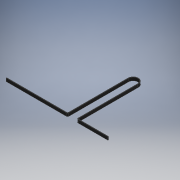
# Autodesk Inventor part: HeaderSliderBelt
Saved by Autodesk Inventor 2017 (Build 210142000, 142)
## iProperties
Created: 2016-12-13
Part Number: HeaderSliderBelt
Material: Rubber
Document SubType Name: Modeling
Designer: umr
Density: 0.93 g/cm^3
Appearance: Rubber - Black
Author: umr
Autodesk Inventor part; units mm, degrees
ref_plane "YZ Plane" through (0, 0, 0) normal (1, 0, 0) x (0, 1, 0)
ref_plane "XZ Plane" through (0, 0, 0) normal (0, 1, 0) x (-1, 0, 0)
ref_plane "XY Plane" through (0, 0, 0) normal (0, 0, 1) x (1, 0, 0)
sketch "Sketch1" plane through (0, 0, 0) normal (0, 0, 1) x (1, 0, 0)
  line L0 (0, 0) -> (99.0465, 0)
  line L1 (98.0465, 0.9998) -> (0.0465, 0.9998)
  line L2 (0.0465, 0.9998) -> (0, 0)
  line L3 (100.0262, 0) -> (101.0465, 0)
  line L4 (101.0465, 2) -> (101.0465, 100)
  line L5 (100.0465, 100) -> (100.0465, 2.9998)
  line L6 (116.9623, 98.8064) -> (116.9623, 3)
  line L7 (116.735, 0) -> (116.0465, 0.7253)
  line L8 (116.0465, 2) -> (116.0465, 100)
  arc A0 (116.9623, 98.8064) -> (100.0465, 100) centre (108.5465, 100) ccw
  arc A1 (116.0465, 100) -> (101.0465, 100) centre (108.5465, 100) ccw
  line L9 (118.0465, 0) -> (166.9623, 0)
  line L10 (166.9623, 0) -> (166.9623, 1)
  line L11 (166.9623, 1) -> (118.9623, 1)
  arc A2 (116.9623, 3) -> (118.9623, 1) centre (118.9623, 3) ccw
  arc A3 (116.0465, 2) -> (118.0465, 0) centre (118.0465, 2) ccw
  arc A4 (98.0465, 0.9998) -> (100.0465, 2.9998) centre (98.0465, 2.9998) ccw
  arc A5 (99.0465, 0) -> (101.0465, 2) centre (99.0465, 2) ccw
  point P0 (100.0465, 0.9998)
  point P1 (116.9623, 1)
  dimension "d0" = 100
  dimension "d1" = 1
  dimension "d2" = 100
  dimension "d3" = 1
  dimension "d4" = 1
  dimension "d6" = 15
  dimension "d7" = 17
  dimension "d8" = 8.5
  dimension "d9" = 15
  dimension "d10" = 50
  dimension "d11" = 1
  dimension "d12" = 2
  dimension "d15" = 100
  constraints: 24 end point, 12 point on circle, 8 point on line, 8 tangent, 6 centre point, 4 parallel, 3 equal radius, 3 horizontal, 2 perpendicular, 1 coincident
  measures "d0" distance of point (100.047, 1) L1.end
  measures "d1" distance of point (100.047, 1) L3.start
  measures "d2" distance of L4.end L3.end
  measures "d3" distance of L5.start L4.end
  measures "d4" distance of L7.start L7.end
  measures "d6" distance between parallel lines of L4 L8
  measures "d7" diameter of A0
  measures "d8" distance from line of A0.centre L5
  measures "d9" diameter of A1
  measures "d10" distance of point (116.962, 1) L10.end
  measures "d11" distance of L10.end L9.end
  measures "d12" radius of A2
  measures "d15" distance from line of A0.centre L9
extrude "Extrusion1" add sketch "Sketch1" along normal blind 5
equation "\"d3\" = d1"
equation "\"d4\" = d3"
equation "\"d15\" = d2"
body "Solid1"
